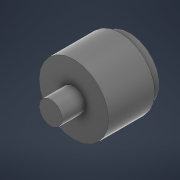
# Autodesk Inventor part: stredne_koleso
Saved by Autodesk Inventor 2022 (Build 260153000, 153)
## iProperties
Created: 2021-12-17
Part Number: stredne_koleso
Material: Generic
Document SubType Name: Modeling
Designer: MatusBarany
Density: 1 g/cm^3
Appearance: Default
Author: MatusBarany
Autodesk Inventor part; units mm, degrees
ref_plane "YZ Plane" through (0, 0, 0) normal (1, 0, 0) x (0, 1, 0)
ref_plane "XZ Plane" through (0, 0, 0) normal (0, 1, 0) x (-1, 0, 0)
ref_plane "XY Plane" through (0, 0, 0) normal (0, 0, 1) x (1, 0, 0)
sketch "Sketch1" plane through (0, 0, 0) normal (0, 0, 1) x (1, 0, 0)
  circle A0 centre (0, 0) radius 7.5
  dimension "d0" = 15
  constraints: 1 centre point, 1 coincident
  measures "d0" diameter of A0
extrude "Extrusion1" add sketch "Sketch1" along normal blind 10
sketch "Sketch2" plane through (0, 0, 0) normal (0, 0, -1) x (-1, 0, 0)
  circle A0 centre (0, 0) radius 6.5
  circle A1 centre (0, 0) radius 5
  circle A2 centre (0, 0) radius 7.5 projected
  dimension "d3" = 13
  dimension "d4" = 15
  dimension "d5" = 10
  constraints: 2 centre point, 2 coincident
  measures "d3" diameter of A0
  measures "d4" diameter of A2
  measures "d5" diameter of A1
extrude "Extrusion2" add sketch "Sketch2" along normal blind 2 contours A0
sketch "Sketch3" plane through (0, 0, 10) normal (0, 0, 1) x (1, 0, 0)
  circle A0 centre (0, 0) radius 7.5 projected
  circle A1 centre (0, 0) radius 2.5
  dimension "d8" = 15
  dimension "d13" = 5
  constraints: 1 centre point
  measures "d8" diameter of A0
  measures "d13" diameter of A1
extrude "Extrusion3" add sketch "Sketch3" along normal blind 5 contours A1
chamfer "Chamfer1" distance 2 angle 68.199 1 edges at (5, 0, 0) measured on face at (-4.9838, -0.4023, -1.3333)
body "Solid1"
